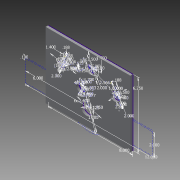
# Autodesk Inventor part: OutlineSketch1
Saved by Autodesk Inventor 2013 (Build 170138000, 138)
## iProperties
Created: 2013-06-03
Part Number: OutlineSketch1
Material: Generic
Document SubType Name: Modeling
Designer: mvarma
Density: 1 g/cm^3
Author: mvarma
Autodesk Inventor part; units mm, degrees
ref_plane "YZ Plane" through (0, 0, 0) normal (1, 0, 0) x (0, 1, 0)
ref_plane "XZ Plane" through (0, 0, 0) normal (0, 1, 0) x (-1, 0, 0)
ref_plane "XY Plane" through (0, 0, 0) normal (0, 0, 1) x (1, 0, 0)
sketch "Sketch1" plane through (0, 0, 0) normal (0, 0, 1) x (1, 0, 0)
  line L0 (0, 0) -> (304.8, 0) construction
  line L1 (304.8, 0) -> (304.8, 50.8) construction
  line L2 (304.8, 50.8) -> (0, 50.8) construction
  line L3 (0, 50.8) -> (0, 0) construction
  circle A0 centre (152.4, 25.4) radius 14.2875
  circle A1 centre (152.4, 25.4) radius 30.48 construction
  circle A2 centre (152.4, 25.4) radius 22.225 construction
  line L4 (152.4, 25.4) -> (138.5082, 62.9697) construction
  circle A3 centre (138.5082, 62.9697) radius 9.525 construction
  circle A4 centre (138.5082, 62.9697) radius 17.78 construction
  circle A5 centre (89.9711, 85.09) radius 31.75
  circle A6 centre (160.9785, 111.3458) radius 31.75
  circle A7 centre (220.6325, 85.09) radius 31.75
  line L5 (0, 50.8) -> (0, 53.34) construction
  line L6 (0, 53.34) -> (304.8, 53.34) construction
  line L7 (304.8, 53.34) -> (304.8, 50.8) construction
  circle A8 centre (138.5082, 62.9697) radius 21.59 construction
  circle A9 centre (152.4, 25.4) radius 46.99 construction
  circle A10 centre (152.4, 25.4) radius 50.8 construction
  arc A11 (84.9408, 79.3264) -> (90.9184, 92.6811) centre (89.9711, 85.09) ccw construction
  circle A12 centre (160.9785, 111.3458) radius 7.65 construction
  circle A13 centre (220.6325, 85.09) radius 7.65 construction
  circle A14 centre (160.9785, 111.3458) radius 9.1 construction
  line L8 (164.8287, 119.5911) -> (223.8692, 92.0215) construction
  line L9 (157.4988, 102.9373) -> (217.7073, 78.0214) construction
  circle A15 centre (138.5082, 62.9697) radius 22.9 construction
  line L10 (84.9408, 79.3264) -> (123.4503, 45.7166) construction
  line L11 (168.5483, 110.2412) -> (161.1682, 59.6633) construction
  line L12 (90.9184, 92.6811) -> (89.9711, 85.09) construction
  line L13 (89.9711, 85.09) -> (84.9408, 79.3264) construction
  circle A16 centre (126.192, 96.2783) radius 3.175
  circle A17 centre (126.192, 96.2783) radius 7.9375 construction
  line L14 (90.9184, 92.6811) -> (125.2091, 88.4019) construction
  line L15 (132.0626, 90.936) -> (155.3205, 116.4945) construction
  line L16 (155.3205, 116.4945) -> (160.9785, 111.3458) construction
  line L17 (168.5483, 110.2412) -> (160.9785, 111.3458) construction
  line L18 (138.5082, 62.9697) -> (126.192, 96.2783) construction
  line L19 (89.9711, 85.09) -> (160.9785, 111.3458) construction
  line L20 (152.4, 25.4) -> (89.9711, 85.09) construction
  line L21 (152.4, 25.4) -> (160.9785, 111.3458) construction
  circle A18 centre (126.192, 96.2783) radius 9.2075 construction
  circle A19 centre (126.192, 96.2783) radius 6.1595 construction
  arc A20 (90.9184, 92.6811) -> (84.9408, 79.3264) centre (89.9711, 85.09) ccw construction
  line L22 (160.9785, 111.3458) -> (220.6325, 85.09) construction
  circle A21 centre (160.9785, 111.3458) radius 25.4 construction
  circle A22 centre (220.6325, 85.09) radius 25.4 construction
  line L23 (102.9424, 114.0695) -> (76.9998, 56.1105) construction
  circle A23 centre (89.9711, 85.09) radius 25.4 construction
  line L24 (209.1281, 114.6824) -> (232.1368, 55.4976) construction
  circle A24 centre (160.9785, 111.3458) radius 10.16
  line L25 (54.4111, 146.9058) -> (257.6111, 146.9058)
  line L26 (257.6111, 146.9058) -> (257.6111, -11.8442)
  line L27 (257.6111, -11.8442) -> (54.4111, -11.8442)
  line L28 (54.4111, -11.8442) -> (54.4111, 146.9058)
  circle A25 centre (138.5082, 62.9697) radius 11.1125
  arc A26 (225.0295, 75.8783) -> (218.6208, 95.1612) centre (221.8252, 85.5197) ccw
  line L29 (219.4627, 84.6013) -> (229.8359, 61.416) construction
  line L30 (221.8252, 85.5197) -> (229.8359, 61.416) construction
  line L31 (219.4627, 84.6013) -> (209.0895, 107.7866) construction
  line L32 (221.8252, 85.5197) -> (213.8144, 109.6234) construction
  arc A27 (208.117, 109.9602) -> (210.062, 105.6129) centre (209.0895, 107.7866) ccw
  arc A28 (214.5654, 107.3637) -> (213.0634, 111.8831) centre (213.8144, 109.6234) ccw
  arc A29 (214.5654, 107.3637) -> (210.062, 105.6129) centre (229.8359, 61.416) ccw
  arc A30 (213.0634, 111.8831) -> (208.117, 109.9602) centre (229.8359, 61.416) ccw
  line L33 (209.0895, 107.7866) -> (208.117, 109.9602) construction
  line L34 (213.8144, 109.6234) -> (213.0634, 111.8831) construction
  arc A31 (218.6208, 95.1612) -> (215.3134, 93.8754) centre (229.8359, 61.416) ccw
  arc A32 (225.0295, 75.8783) -> (223.612, 75.3272) centre (229.8359, 61.416) ccw
  line L35 (102.6358, 107.1803) -> (91.1149, 84.5434) construction
  line L36 (79.5941, 61.9064) -> (88.8014, 85.5789) construction
  arc A33 (98.8719, 111.4706) -> (97.1455, 107.0321) centre (98.0087, 109.2513) ccw
  arc A34 (101.5557, 105.0581) -> (103.7158, 109.3025) centre (102.6358, 107.1803) ccw
  arc A35 (101.5557, 105.0581) -> (97.1455, 107.0321) centre (79.5941, 61.9064) ccw
  line L37 (98.0087, 109.2513) -> (98.8719, 111.4706) construction
  line L38 (102.6358, 107.1803) -> (103.7158, 109.3025) construction
  arc A36 (103.7158, 109.3025) -> (98.8719, 111.4706) centre (79.5941, 61.9064) ccw
  arc A37 (215.3134, 93.8754) -> (223.612, 75.3272) centre (219.4627, 84.6013) ccw
  arc A38 (86.5066, 75.4886) -> (95.7233, 93.5981) centre (91.1149, 84.5434) ccw
  line L39 (88.8014, 85.5789) -> (98.0087, 109.2513) construction
  line L40 (91.1149, 84.5434) -> (79.5941, 61.9064) construction
  arc A39 (86.5066, 75.4886) -> (85.1185, 76.1099) centre (79.5941, 61.9064) ccw
  arc A40 (95.7233, 93.5981) -> (92.4843, 95.0479) centre (79.5941, 61.9064) ccw
  arc A41 (92.4843, 95.0479) -> (85.1185, 76.1099) centre (88.8014, 85.5789) ccw
  line L41 (160.9785, 111.3458) -> (137.7306, 121.5779) construction
  point P0 (184.2263, 101.1136)
  point P1 (211.429, 108.764)
  point P2 (100.3481, 108.2736)
  dimension "d1" = 50.8
  dimension "d2" = 28.575
  dimension "d3" = 25.4
  dimension "d4" = 152.4
  dimension "d7" = 60.96
  dimension "d8" = 44.45
  dimension "d9" = 19.05
  dimension "d10" = 35.56
  dimension "d11" = 40.0558
  dimension "d12" = 63.5
  dimension "d13" = 63.5
  dimension "d14" = 63.5
  dimension "d15" = 2.54
  dimension "d16" = 304.8
  dimension "d17" = 43.18
  dimension "d18" = 93.98
  dimension "d19" = 101.6
  dimension "d21" = 15.3
  dimension "d22" = 15.3
  dimension "d23" = 15.3
  dimension "d24" = 18.2
  dimension "d29" = 45.8
  dimension "d30" = 146
  dimension "d31" = 6.35
  dimension "d32" = 15.875
  dimension "d33" = 146
  dimension "d35" = 18.415
  dimension "d37" = 12.319
  dimension "d38" = 65.1764
  dimension "d40" = 50.8
  dimension "d41" = 50.8
  dimension "d42" = 17
  dimension "d43" = 17
  dimension "d44" = 50.8
  dimension "d45" = 45
  dimension "d50" = 20.32
  dimension "d53" = 203.2
  dimension "d54" = 158.75
  dimension "d55" = 35.56
  dimension "d56" = 35.56
  dimension "d57" = 22.225
  dimension "d67" = 25.4
  dimension "d68" = 25.4
  dimension "d69" = 2.86
  dimension "d70" = 25.4
  dimension "d71" = 25.4
  dimension "d72" = 4.7625
  dimension "d75" = 2.86
  dimension "d80" = 4.7625
  dimension "d82" = 4.7625
  dimension "d83" = 50.8
  dimension "d84" = 50.8
  dimension "d85" = 10.16
  dimension "d97" = 48.4188
  dimension "d99" = 20.32
  dimension "d101" = 25.4
  dimension "d102" = 25.4
  dimension "d103" = 10.16
  dimension "d104" = 180
  constraints: 86 end point, 57 point on circle, 42 centre point, 31 coincident, 16 tangent, 14 point on line, 9 collinear, 7 perpendicular, 5 parallel, 2 horizontal, 2 midpoint, 1 equal radius, 3 other
  measures "d1" distance of L1.end L0.end
  measures "d2" diameter of A0
  measures "d3" distance from line of L0 A0.centre
  measures "d4" distance from line of L3 A0.centre
  measures "d7" diameter of A1
  measures "d8" diameter of A2
  measures "d9" diameter of A3
  measures "d10" diameter of A4
  measures "d11" distance of L4.start L4.end
  measures "d12" diameter of A5
  measures "d13" diameter of A6
  measures "d14" diameter of A7
  measures "d15" distance of L2.end L5.end
  measures "d16" distance of L0.end L0.start
  measures "d17" diameter of A8
  measures "d18" diameter of A9
  measures "d19" diameter of A10
  measures "d21" diameter of A11
  measures "d22" diameter of A12
  measures "d23" diameter of A13
  measures "d24" diameter of A14
  measures "d29" diameter of A15
  measures "d30" angle of L13 L12
  measures "d31" diameter of A16
  measures "d32" diameter of A17
  measures "d33" angle of L17 L16
  measures "d35" diameter of A18
  measures "d37" diameter of A19
  measures "d38" distance of L22.end L16.end
  measures "d40" diameter of A21
  measures "d41" diameter of A22
  measures "d42" angle of L12 L23
  measures "d43" angle of L13 L23
  measures "d44" diameter of A23
  measures "d45" angle of L22 L24
  measures "d50" diameter of A24
  measures "d53" distance of L26.end L27.end
  measures "d54" distance of L25.end L26.end
  measures "d55" distance from line of L28 A5.centre
  measures "d56" distance from line of L25 A6.centre
  measures "d57" diameter of A25
  measures "d67" distance of L29.start L29.end
  measures "d68" distance of L30.start L29.end
  measures "d69" angle of L24 L29
  measures "d70" distance of L29.start L31.end
  measures "d71" distance of L30.start L32.end
  measures "d72" diameter of A27
  measures "d75" angle of L23 L35
  measures "d80" diameter of A33
  measures "d82" diameter of A34
  measures "d83" distance of L36.start L39.end
  measures "d84" distance of L35.start L36.start
  measures "d85" radius of A26
  measures "d97" radius of A35
  measures "d99" diameter of A38
  measures "d101" distance of L36.start L36.end
  measures "d102" distance of L35.end L36.start
  measures "d103" radius of A41
  measures "d104" angle of L22 L41
extrude "Extrusion2" add sketch "Sketch1" along normal blind 6.35 contours A5 | A6 | A7 | L25 L26 L27 L28
hole "Hole2" at (79.5941, 61.9064, 0) at (229.8359, 61.416, 0) at (184.2263, 101.1136, 0) at (137.7306, 121.5779, 0) direction (0, 0, 1) diameter 4.7625 end through all
equation "\"d2\" = BearingLargeOD"
equation "\"d7\" = Gear48tPD"
equation "\"d8\" = Gear35tPD"
equation "\"d9\" = Gear15tPD"
equation "\"d10\" = Gear28tPD"
equation "\"d11\" = 0.5 * Gear48tPD + 0.5 * Gear15tPD + MeshingClearance"
equation "\"d12\" = CimOD"
equation "\"d13\" = CimOD"
equation "\"d14\" = CimOD"
equation "\"d17\" = Gear28tPD + ClearanceDiameter"
equation "\"d18\" = WheelOD"
equation "\"d19\" = WheelClearance"
equation "\"Pulley48tPD\" = 45.8"
equation "\"Pulley19tPD\" = 18.2"
equation "\"Pulley16tPD\" = 15.3"
equation "\"Gear15tPD\" = 19.05"
equation "\"Gear35tPD\" = 44.45"
equation "\"Gear48tPD\" = 60.96"
equation "\"Gear28tPD\" = 35.56"
equation "\"BearingLargeOD\" = 28.575"
equation "\"BearingSmallOD\" = 22.225"
equation "\"MeshingClearance\" = 0.0508"
equation "\"CimOD\" = 63.5"
equation "\"WheelOD\" = 93.98"
equation "\"ClearanceDiameter\" = 7.62"
equation "\"WheelClearance\" = 101.6"
equation "\"TensioningBearingID\" = 6.35"
equation "\"TensioningBearingOD\" = 15.875"
equation "\"SpingClipClearance\" = 8.89"
equation "\"Pi\" = 79.79645"
body "Solid2"
